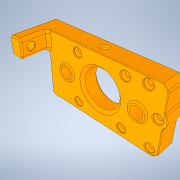
# Autodesk Inventor part: Кронштейн тянущего шаговика
Saved by Autodesk Inventor 2021.1 (Build 251245010, 245A)
## iProperties
Created: 2026-05-18
Part Number: Кронштейн тянущего шаговика
Material: Типовые
Document SubType Name: Modeling
Designer: Андрей Тарасов
Density: 1 g/cm^3
Appearance: По умолчанию
Author: Андрей Тарасов
Autodesk Inventor part; units mm, degrees
ref_plane "YZ Plane" through (0, 0, 0) normal (1, 0, 0) x (0, 1, 0)
ref_plane "XZ Plane" through (0, 0, 0) normal (0, 1, 0) x (-1, 0, 0)
ref_plane "XY Plane" through (0, 0, 0) normal (0, 0, 1) x (1, 0, 0)
sketch "Эскиз1" plane through (0, 0, 0) normal (0, 0, 1) x (1, 0, 0)
  line L0 (38, -21) -> (-38, -21)
  line L1 (-38, -21) -> (-38, 21)
  line L2 (-38, 21) -> (38, 21)
  line L3 (38, 21) -> (38, -21)
  line L4 (38, -21) -> (-38, 21) construction
  line L5 (-38, -21) -> (38, 21) construction
  line L6 (-38, 0) -> (38, 0) construction
  circle A0 centre (-24, 0) radius 4
  circle A1 centre (24, 0) radius 4
  circle A2 centre (0, 0) radius 12
  line L7 (21, 21) -> (21, -21) construction
  line L8 (28, -21) -> (28, 21) construction
  circle A3 centre (33, -17) radius 1.6
  circle A4 centre (28, 17) radius 1.6
  line L9 (38, 2) -> (-38, 2) construction
  circle A5 centre (35, 2) radius 1.6
  line L10 (15.5, -15.5) -> (-15.5, -15.5) construction
  line L11 (-15.5, -15.5) -> (-15.5, 15.5) construction
  line L12 (-15.5, 15.5) -> (15.5, 15.5) construction
  line L13 (15.5, 15.5) -> (15.5, -15.5) construction
  line L14 (15.5, -15.5) -> (-15.5, 15.5) construction
  line L15 (-15.5, -15.5) -> (15.5, 15.5) construction
  circle A6 centre (-15.5, 15.5) radius 1.6
  circle A7 centre (15.5, 15.5) radius 1.6
  circle A8 centre (15.5, -15.5) radius 1.6
  circle A9 centre (-15.5, -15.5) radius 1.6
  arc A10 (38, 6) -> (38, -2) centre (35, 2) ccw construction
  arc A11 (38, -2) -> (38, 6) centre (35, 2) ccw
  point P0 (38, 5)
  point P1 (38, -3)
  dimension "d1" = 8
  dimension "d2" = 24
  dimension "d3" = 24
  dimension "d4" = 76
  dimension "d5" = 42
  dimension "d8" = 24
  dimension "d13" = 17
  dimension "d14" = 7
  dimension "d17" = 3.2
  dimension "d31" = 3
  dimension "d37" = 31
  dimension "d40" = 4
  dimension "d42" = 10
  dimension "d82" = 5
  dimension "d84" = 34
  dimension "d94" = 19
  constraints: 32 end point, 12 centre point, 12 point on line, 7 equal radius, 6 coincident, 6 midpoint, 6 perpendicular, 4 parallel, 4 point on circle, 2 horizontal
  measures "d1" diameter of A1
  measures "d2" distance of point (0, 0) A0.centre
  measures "d3" distance of A1.centre point (0, 0)
  measures "d4" distance between parallel lines of L3 L1
  measures "d5" distance of L0.end L1.end
  measures "d8" diameter of A2
  measures "d13" distance between parallel lines of L3 L7
  measures "d14" distance between parallel lines of L8 L7
  measures "d17" diameter of A3
  measures "d31" distance from line of L3 A5.centre
  measures "d37" distance of L11.end L12.end
  measures "d40" distance from line of L0 A3.centre
  measures "d42" diameter of A10
  measures "d82" distance from line of A3.centre L8
  measures "d84" vertical distance of A4.centre A3.centre
  measures "d94" distance from line of A3.centre L9
extrude "Выдавливание1" add sketch "Эскиз1" along normal blind 12
sketch "Эскиз2" plane through (0, 0, 12) normal (0, 0, 1) x (1, 0, 0)
  circle A0 centre (-24, 0) radius 4 projected
  circle A1 centre (24, 0) radius 4 projected
  circle A2 centre (-24, 0) radius 5
  circle A3 centre (24, 0) radius 4 projected
  circle A4 centre (24, 0) radius 5
  point P0 (0, 0)
  dimension "d9" = 10
  constraints: 2 centre point, 2 coincident, 1 equal radius
  measures "d9" diameter of A2
extrude "Выдавливание2" add sketch "Эскиз2" along normal blind 1
sketch "Эскиз4" plane through (0, 0, 0) normal (0, 0, -1) x (-1, 0, 0)
  circle A0 centre (-24, 0) radius 4 construction
  circle A1 centre (24, 0) radius 4 construction
  circle A2 centre (-24, 0) radius 4 construction
  line L0 (-21.6906, 4) -> (-19.3812, 0)
  line L1 (-19.3812, 0) -> (-21.6906, -4)
  line L2 (-21.6906, -4) -> (-26.3094, -4)
  line L3 (-26.3094, -4) -> (-28.6188, 0)
  line L4 (-28.6188, 0) -> (-26.3094, 4)
  line L5 (-26.3094, 4) -> (-21.6906, 4)
  circle A3 centre (24, 0) radius 4 construction
  line L6 (21.6906, 4) -> (26.3094, 4)
  line L7 (26.3094, 4) -> (28.6188, 0)
  line L8 (28.6188, 0) -> (26.3094, -4)
  line L9 (26.3094, -4) -> (21.6906, -4)
  line L10 (21.6906, -4) -> (19.3812, 0)
  line L11 (19.3812, 0) -> (21.6906, 4)
  point P0 (0, 0)
  dimension "d22" = 8
  dimension "d23" = 8
  constraints: 24 end point, 2 coincident, 1 collinear, 26 other
  measures "d22" distance between parallel lines of L2 L5
  measures "d23" distance between parallel lines of L9 L6
extrude "Выдавливание3" cut sketch "Эскиз4" against normal blind 4.5
sketch "Эскиз5" plane through (0, 0, 12) normal (0, 0, 1) x (1, 0, 0)
  circle A0 centre (33, -17) radius 1.6 projected
  circle A1 centre (33, -17) radius 2.8
  circle A2 centre (28, 17) radius 1.6 projected
  circle A3 centre (28, 17) radius 2.8
  circle A4 centre (35, 2) radius 1.6 projected
  circle A5 centre (35, 2) radius 2.8
  circle A6 centre (-15.5, 15.5) radius 1.6 projected
  circle A7 centre (-15.5, 15.5) radius 2.8
  circle A8 centre (15.5, 15.5) radius 1.6 projected
  circle A9 centre (15.5, 15.5) radius 2.8
  circle A10 centre (-15.5, -15.5) radius 1.6 projected
  circle A11 centre (-15.5, -15.5) radius 2.8
  circle A12 centre (15.5, -15.5) radius 1.6 projected
  circle A13 centre (15.5, -15.5) radius 2.8
  point P0 (0, 0)
  dimension "d27" = 5.6
  constraints: 7 centre point, 7 coincident, 6 equal radius
  measures "d27" diameter of A1
extrude "Выдавливание4" cut sketch "Эскиз5" against normal blind 2 contours A0 | A1 | A2 | A3 | A4 | A5 | A6 | A7 | A8 | A9 | A10 | A11 | A12 | A13
chamfer "Фаска1" distance 3 angle 45 2 edges at (38, 21, 6) (38, -21, 6)
sketch "Эскиз7" plane through (-38, -21, 0) normal (-1, 0, 0) x (0, 0, 1)
  line L0 (0, 42) -> (12, 42) projected
  line L1 (0, 42) -> (30, 42)
  line L2 (30, 42) -> (30, 30)
  line L3 (30, 30) -> (0, 30)
  line L4 (0, 30) -> (0, 42)
  circle A0 centre (23.7, 36) radius 3
  line L5 (0, 42) -> (0, 0) projected
  line L6 (12, 33) -> (12, 9) construction
  line L7 (-14, 21) -> (35, 21) construction
  point P0 (0, 21)
  point P1 (12, 21)
  dimension "d51" = 6
  dimension "d54" = 30
  dimension "d55" = 12
  dimension "d56" = 11.7
  dimension "d57" = 15
  constraints: 10 end point, 2 horizontal, 2 parallel, 1 centre point, 1 midpoint, 1 perpendicular, 1 point on line
  measures "d51" diameter of A0
  measures "d54" distance between parallel lines of L2 L4
  measures "d55" distance of L3.end L0.start
  measures "d56" distance from line of A0.centre L6
  measures "d57" distance from line of L7 A0.centre
extrude "Выдавливание6" add sketch "Эскиз7" along normal blind 9
sketch "Эскиз8" plane through (-38, -21, 0) normal (1, 0, 0) x (0, 0, -1)
  circle A0 centre (-23.7, 36) radius 3 projected
  circle A1 centre (-23.7, 36) radius 2.5
  point P0 (0, 21)
  dimension "d60" = 5
  constraints: 1 centre point, 1 coincident
  measures "d60" diameter of A1
extrude "Выдавливание7" add sketch "Эскиз8" against normal blind 1
fillet "Сопряжение1" radius 2 9 edges at (-38, 9, 21) (-38, 21, 21) (-47, 21, 15) (-47, 9, 15) (-38, 9, 6) (-38, -21, 6) (38, -2, 6) (38, 6, 6) (38, 18, 6)
chamfer "Фаска3" distance 2 angle 45 5 edges at (-12, 0, 0) (-12, 0, 12) (-38, 15, 12) (-38.5858, 9.5858, 12) (-38.5858, 20.4142, 12)
chamfer "Фаска4" distance 0.4 angle 45 40 edges at (-38, -6, 12) (-37.4142, -20.4142, 12) (-0.5, -21, 12) (-38.0159, 7.252, 12) (38, 12.0353, 12) (37.8478, 17.9369, 12) (36.2071, 19.7929, 12) (38.1484, 6.1431, 12) (40, 2, 12) (38.1484, -2.1431, 12) (38, -10.4495, 12) (-0.7679, 21, 12) (-0.5, -21, 0) (-37.4142, -20.4142, 0) (-38, -6, 0) (-38.5858, 8.4142, 0) (-42.5, 9, 0) (-46.4142, 9.5858, 0) (-47, 15, 0) (-46.4142, 20.4142, 0) (-5, 21, 0) (38, 12.0353, 0) (37.8478, 17.9369, 0) (36.2071, 19.7929, 0) (38.1484, 6.1431, 0) (40, 2, 0) (38.1484, -2.1431, 0) (38, -10.4495, 0) (25.2, 17, 12) (32.2, 2, 12) (30.2, -17, 12) (31.4, -17, 0) (33.4, 2, 0) (26.4, 17, 0) (-18.3, 15.5, 12) (12.7, 15.5, 12) (-18.3, -15.5, 12) (12.7, -15.5, 12) (36.5, -19.5, 12) (36.5, -19.5, 0)
chamfer "Фаска5" distance 1 angle 45 8 edges at (-47, 15, 30) (-46.4142, 20.4142, 30) (-42.5, 21, 30) (-38.5858, 20.4142, 30) (-38, 15, 30) (-38.5858, 9.5858, 30) (-42.5, 9, 30) (-46.4142, 9.5858, 30)
fillet "Сопряжение2" radius 0.4 3 edges at (-39, 15, 26.2) (-38, 15, 26.2) (-47, 15, 20.7)
fillet "Сопряжение3" radius 0.8 12 edges at (-26.3094, -4, 2.25) (-21.6906, -4, 2.25) (-19.3812, 0, 2.25) (-28.6188, 0, 2.25) (-26.3094, 4, 2.25) (-21.6906, 4, 2.25) (19.3812, 0, 2.25) (21.6906, 4, 2.25) (21.6906, -4, 2.25) (26.3094, -4, 2.25) (28.6188, 0, 2.25) (26.3094, 4, 2.25)
chamfer "Фаска6" distance 0.6 angle 45 24 edges at (24, -4, 0) (26.2475, -3.8928, 0) (27.4641, -2, 0) (28.495, 0, 0) (27.4641, 2, 0) (26.2475, 3.8928, 0) (24, 4, 0) (21.7525, 3.8928, 0) (20.5359, 2, 0) (19.505, 0, 0) (20.5359, -2, 0) (21.7525, -3.8928, 0) (-24, -4, 0) (-21.7525, -3.8928, 0) (-20.5359, -2, 0) (-19.505, 0, 0) (-20.5359, 2, 0) (-21.7525, 3.8928, 0) (-24, 4, 0) (-26.2475, 3.8928, 0) (-27.4641, 2, 0) (-28.495, 0, 0) (-27.4641, -2, 0) (-26.2475, -3.8928, 0)
chamfer "Фаска7" distance 1.2 angle 45 7 edges at (-18.3, 15.5, 10) (12.7, 15.5, 10) (25.2, 17, 10) (32.2, 2, 10) (-18.3, -15.5, 10) (12.7, -15.5, 10) (30.2, -17, 10)
chamfer "Фаска8" distance 1 angle 45 2 edges at (-29, 0, 12) (19, 0, 12)
sketch "Эскиз9" plane through (-45, 21, 0.4) normal (0, 1, 0) x (1, 0, 0)
  line L0 (0, -5.6) -> (80, -5.6) construction
  line L1 (80, 0) -> (80, -11.2) projected
  line L2 (0, -28.6) -> (0, 0) projected
  circle A0 centre (42, -5.6) radius 2
  line L3 (83, -11.2) -> (83, 0) projected
  point P0 (45, 0.4)
  dimension "d89" = 4
  dimension "d90" = 41
  constraints: 2 end point, 2 point on line, 1 centre point, 1 horizontal, 1 midpoint
  measures "d89" diameter of A0
  measures "d90" distance from line of L3 A0.centre
extrude "Выдавливание8" cut sketch "Эскиз9" against normal blind 6
fillet "Сопряжение4" radius 1 1 edges at (-5, 21, 6)
equation "\"d3\" = d2"
equation "\"d20\" = d18"
equation "\"d18\" = 4"
